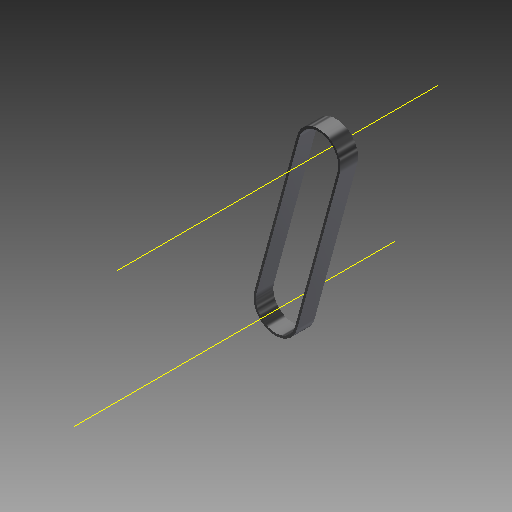
# Autodesk Inventor part: Synchronous Belt
Saved by Autodesk Inventor 2017 SP1 (Build 210196100, 196)
## iProperties
Created: 2017-05-14
Part Number: Synchronous Belt
Material: Rubber
Document SubType Name: Modeling
Designer: Zach
Density: 1 g/cm^3
Appearance: Rubber - Black - Version 1.1
CustomPartVersion: 1
Author: Zach
Autodesk Inventor part; units mm, degrees
sketch "Sketch Path" plane through (0, 0, 0) normal (0, 0, 1) x (1, 0, 0)
  arc A0 (-25.2482, 5.4864) -> (11.5925, -4.6025) centre (-6.8278, 0.442) ccw
  arc A1 (50.5673, 137.717) -> (13.7266, 147.8059) centre (32.1469, 142.7615) ccw
  line L0 (50.5673, 137.717) -> (11.5925, -4.6025)
  line L1 (-25.2482, 5.4864) -> (13.7266, 147.8059)
  constraints: 4 end point, 4 point on circle, 2 centre point
ref_plane "Cross Section Plane" through (11.5925, -4.6025, 0) normal (0.2641, 0.9645, 0) x (0, 0, 1)
ref_plane "Work Plane2" through (-6.8278, 0.442, 0) normal (0.866, 0.5, 0) x (0, 0, 1)
ref_plane "Work Plane3" through (32.1469, 142.7615, 0) normal (-0.6063, -0.7953, 0) x (0, 0, 1)
sketch "Cross Section" plane through (11.5925, -4.6025, 0) normal (0.2641, 0.9645, 0) x (0, 0, 1)
  line L0 (-8, 1) -> (8, 1)
  line L1 (8, 1) -> (8, -1)
  line L2 (8, -1) -> (-8, -1)
  line L3 (-8, -1) -> (-8, 1)
  line L4 (-8, 0) -> (8, 0) construction
  point P0 (0, 0)
  point P1 (0, 0)
  dimension "d0" = 16
  dimension "d4" = 1
  dimension "d5" = 1
  constraints: 10 end point, 3 midpoint, 2 parallel, 1 coincident, 1 horizontal, 1 perpendicular, 1 other
  measures "d0" distance between parallel lines of L1 L3
  measures "d4" distance between parallel lines of L2 L4
  measures "d5" distance between parallel lines of L4 L0
sweep "Belt" add profiles "Cross Section" path "Sketch Path"
equation "\"d0\" = da_B"
equation "\"d4\" = da_a"
equation "\"d5\" = da_a2"
equation "\"da_B\" = 16"
equation "\"da_L\" = 415.11945"
equation "\"da_a\" = 1"
equation "\"da_S\" = 5.3"
equation "\"da_Beta\" = 20deg"
equation "\"da_Ht\" = 2.5"
equation "\"da_H\" = 4.5"
equation "\"da_a2\" = 1"
body "Solid1"
